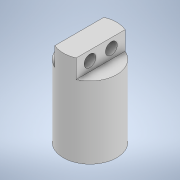
# Autodesk Inventor part: drive_shaft_v4
Saved by Autodesk Inventor 2022 (Build 260153000, 153)
## iProperties
Created: 2022-06-04
Part Number: drive_shaft_v4
Material: Generic
Document SubType Name: Modeling
Designer: kylem
Density: 1 g/cm^3
Appearance: Default
Author: kylem
Autodesk Inventor part; units mm, degrees
ref_plane "YZ Plane" through (0, 0, 0) normal (1, 0, 0) x (0, 1, 0)
ref_plane "XZ Plane" through (0, 0, 0) normal (0, 1, 0) x (-1, 0, 0)
ref_plane "XY Plane" through (0, 0, 0) normal (0, 0, 1) x (1, 0, 0)
sketch "Sketch1" plane through (0, 0, 0) normal (0, 1, 0) x (-1, 0, 0)
  circle A0 centre (0, 0) radius 5
  dimension "d0" = 10
  constraints: 1 centre point, 1 coincident
  measures "d0" diameter of A0
extrude "Extrusion1" add sketch "Sketch1" along normal blind 17
sketch "Sketch2" plane through (0, 17, 0) normal (0, 1, 0) x (1, 0, 0)
  line L0 (0, 0) -> (-2, 0)
  line L1 (-2, 0) -> (-2, 7.2521)
  line L2 (0, 0) -> (2, 0)
  line L3 (2, 0) -> (2, -7.0492)
  line L4 (2, -7.0492) -> (-2, -7.0492)
  line L5 (-2, -7.0492) -> (-2, 7.2521)
  line L6 (-2, 7.2521) -> (2, 7.2521)
  line L7 (2, 7.2521) -> (2, -7.0492)
  line L8 (-2, -7.0492) -> (-8.2773, -7.0492)
  line L9 (-8.2773, -7.0492) -> (-8.2773, 7.6578)
  line L10 (-8.2773, 7.6578) -> (-2, 7.6578)
  line L11 (-2, 7.6578) -> (-2, -7.0492)
  line L12 (2, 7.2521) -> (6.5688, 7.2521)
  line L13 (6.5688, 7.2521) -> (6.5688, -6.4823)
  line L14 (6.5688, -6.4823) -> (2, -6.4823)
  line L15 (2, -6.4823) -> (2, 7.2521)
  dimension "d3" = 2
  dimension "d4" = 2
  constraints: 32 end point, 6 parallel, 5 horizontal, 5 perpendicular
  measures "d3" distance of L0.start L0.end
  measures "d4" distance of L0.start L2.end
extrude "Extrusion2" cut sketch "Sketch2" against normal blind 3.5 contours L5 L8 L9 L10 L11 L1 | L7 L12 L13 L14 L3
sketch "Sketch3" plane through (2, 17, 4.5826) normal (1, 0, 0) x (0, 0, -1)
  line L0 (9.1652, 0) -> (0, 0) projected
  line L1 (4.5826, 0) -> (4.5826, -1.75)
  line L2 (4.5826, -1.75) -> (2.5826, -1.75)
  line L3 (4.5826, -1.75) -> (6.5826, -1.75)
  circle A0 centre (2.5826, -1.75) radius 1.1
  circle A1 centre (6.5826, -1.75) radius 1.1
  point P0 (4.5826, -17)
  dimension "d7" = 1.75
  dimension "d8" = 2
  dimension "d9" = 2
  dimension "d10" = 2.2
  dimension "d11" = 2.2
  constraints: 6 end point, 2 centre point, 2 coincident, 1 horizontal, 1 midpoint, 1 perpendicular, 1 vertical
  measures "d7" distance of L1.start L1.end
  measures "d8" distance of L1.end L2.end
  measures "d9" distance of L1.end L3.end
  measures "d10" diameter of A0
  measures "d11" diameter of A1
extrude "Extrusion3" cut sketch "Sketch3" against normal blind 56
body "Solid1"
